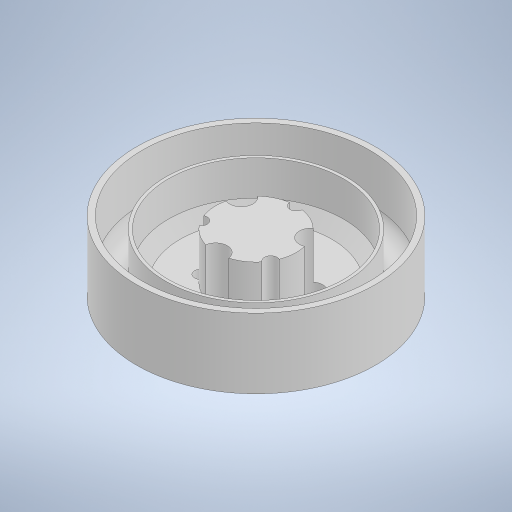
# Autodesk Inventor part: Weapon Mold
Saved by Autodesk Inventor 2023.2 (Build 272271000, 271)
## iProperties
Created: 2023-03-10
Part Number: Weapon Mold
Material: Generic
Document SubType Name: Modeling
Designer: Nathan Cai
Density: 1 g/cm^3
Appearance: Default
Author: Nathan Cai
Autodesk Inventor part; units mm, degrees
ref_plane "YZ Plane" through (0, 0, 0) normal (1, 0, 0) x (0, 1, 0)
ref_plane "XZ Plane" through (0, 0, 0) normal (0, 1, 0) x (-1, 0, 0)
ref_plane "XY Plane" through (0, 0, 0) normal (0, 0, 1) x (1, 0, 0)
sketch "Sketch7" plane through (0, 0, 0) normal (0, 0, 1) x (1, 0, 0)
  line L0 (0, 0) -> (23.8125, 0)
  line L1 (23.8125, 0) -> (23.8125, 12.7)
  line L2 (23.8125, 12.7) -> (0, 12.7) construction
  line L3 (0, 12.7) -> (0, 0)
  line L4 (23.8125, 0) -> (24.6062, 0)
  line L5 (24.6062, 0) -> (24.6062, 12.7)
  line L6 (24.6062, 12.7) -> (23.8125, 12.7)
  line L7 (23.8125, 12.7) -> (23.8125, 0)
  line L8 (30.9562, 0) -> (32.5437, 0)
  line L9 (32.5437, 0) -> (32.5437, 15.875)
  line L10 (32.5437, 15.875) -> (30.9562, 15.875)
  line L11 (30.9562, 15.875) -> (30.9562, 0)
  line L12 (0, 0) -> (32.5437, 0)
  line L13 (32.5437, 0) -> (32.5437, -3.175)
  line L14 (32.5437, -3.175) -> (0, -3.175)
  line L15 (0, -3.175) -> (0, 0)
  line L16 (0, 0) -> (6.35, 0)
  line L17 (6.35, 0) -> (6.35, 19.05)
  line L18 (6.35, 19.05) -> (0, 19.05)
  line L19 (0, 19.05) -> (0, 0)
  line L20 (23.8125, 0) -> (20.6375, 0)
  line L21 (20.6375, 0) -> (20.6375, 1.5875) construction
  line L22 (20.6375, 1.5875) -> (23.8125, 1.5875)
  line L23 (23.8125, 1.5875) -> (23.8125, 0)
  line L24 (20.6375, 0) -> (22.225, 1.5875)
  line L25 (20.6375, 0) -> (22.8826, 0) construction
  point P0 (30.9562, 0)
  point P1 (24.6062, 0)
  point P2 (23.8125, 1.5875)
  point P3 (20.6375, 0)
  point P4 (20.6375, 0)
  dimension "d37" = 23.8125
  dimension "d38" = 12.7
  dimension "d39" = 0.7937
  dimension "d40" = 12.7
  dimension "d41" = 1.5875
  dimension "d42" = 15.875
  dimension "d43" = 6.35
  dimension "d44" = 3.175
  dimension "d45" = 6.35
  dimension "d46" = 19.05
  dimension "d52" = 1.5875
  dimension "d53" = 20.6375
  dimension "d72" = 45
  constraints: 52 end point, 12 parallel, 7 horizontal, 6 perpendicular, 2 point on line, 1 equal length, 1 midpoint
  measures "d37" distance of L2.end L1.end
  measures "d38" distance of L1.end L0.end
  measures "d39" distance of L6.end L5.end
  measures "d40" distance of L5.end L4.end
  measures "d41" distance of L10.end L9.end
  measures "d42" distance of L9.end L8.end
  measures "d43" distance between parallel lines of L11 L5
  measures "d44" distance of L12.end L13.end
  measures "d45" distance of L18.end L17.end
  measures "d46" distance of L17.end L16.end
  measures "d52" distance of L20.end L21.end
  measures "d53" distance between parallel lines of L3 L21
  measures "d72" angle of L25 L24
revolve "Revolution1" add sketch "Sketch7" angle 360 about axis through (0, 19.05, 0) along (0, -1, 0) contours L0 L4 L12 L8 L13 L14 L15 | L24 L22 L1 L0 | L1 L6 L5 L4 | L8 L11 L10 L9
fillet "Fillet1" radius 3.175 2 edges at (-30.9562, 0, 0) (-24.6062, 0, 0)
chamfer "Chamfer4" distance 1.5875 angle 45 1 edges at (-23.8125, 1.5875, 0)
sketch "Sketch8" plane through (0, 0, 0) normal (0, 1, 0) x (1, 0, 0)
  circle A0 centre (0, 0) radius 11 construction
  line L0 (0, 0) -> (0, 11) construction
  circle A1 centre (0, 11) radius 1.7272
  circle A2 centre (-9.5263, -5.5) radius 1.7272
  circle A3 centre (9.5263, -5.5) radius 1.7272
  circle A4 centre (0, -11) radius 3.175
  circle A5 centre (9.5263, 5.5) radius 3.175
  circle A6 centre (-9.5263, 5.5) radius 3.175
  circle A7 centre (0, 0) radius 11
  point P0 (3.1418, -10.5418)
  point P1 (8.5479, -6.9234)
  point P2 (10.2698, -3.941)
  point P3 (10.7003, 2.55)
  point P4 (7.5586, 7.9917)
  point P5 (1.7219, 10.8644)
  point P6 (-1.7219, 10.8644)
  point P7 (-7.5586, 7.9917)
  point P8 (-10.7003, 2.55)
  point P9 (-10.2698, -3.941)
  point P10 (-8.5479, -6.9234)
  point P11 (-3.1418, -10.5418)
  dimension "d57" = 22
  dimension "d58" = 3.4544
  dimension "d61" = 360
  dimension "d63" = 6.35
  dimension "d66" = 360
  constraints: 7 centre point, 3 coincident, 2 end point, 2 point on circle, 1 point on line, 1 vertical, 17 other
  measures "d57" diameter of A0
  measures "d58" diameter of A1
  measures "d63" diameter of A4
extrude "Extrusion7" add sketch "Sketch8" along normal blind 12.7 contours A1 A7 A5 A3 A4 A2 A6
extrude "Extrusion8" cut sketch "Sketch8" against normal through all contours A1 A7 | A7 A1 | A7 A6 | A6 A7 | A7 A5 | A5 A7 | A7 A2 | A2 A7 | A7 A3 | A3 A7 | A7 A4 | A4 A7
body "Solid2"
